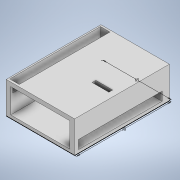
# Autodesk Inventor part: rpi case 4
Saved by Autodesk Inventor 2022.1 (Build 261234020, 234B)
## iProperties
Created: 2022-01-29
Part Number: rpi case 4
Material: Generic
Document SubType Name: Modeling
Designer: 46734
Density: 1 g/cm^3
Appearance: Default
Author: 46734
Autodesk Inventor part; units mm, degrees
ref_plane "YZ Plane" through (0, 0, 0) normal (1, 0, 0) x (0, 1, 0)
ref_plane "XZ Plane" through (0, 0, 0) normal (0, 1, 0) x (-1, 0, 0)
ref_plane "XY Plane" through (0, 0, 0) normal (0, 0, 1) x (1, 0, 0)
sketch "Sketch1" plane through (0, 0, 0) normal (0, 1, 0) x (-1, 0, 0)
  line L0 (32.5, 45) -> (-32.5, 45)
  line L1 (-32.5, 45) -> (-32.5, -45)
  line L2 (-32.5, -45) -> (32.5, -45)
  line L3 (32.5, -45) -> (32.5, 45)
  line L4 (32.5, 45) -> (-32.5, -45) construction
  line L5 (-32.5, 45) -> (32.5, -45) construction
  point P0 (0, 0)
  dimension "d0" = 65
  dimension "d1" = 90
  constraints: 12 end point, 2 midpoint, 2 parallel, 1 horizontal, 1 perpendicular
  measures "d0" distance of L2.end L1.end
  measures "d1" distance of L1.end L0.end
extrude "Extrusion1" add sketch "Sketch1" along normal blind 30
sketch "Sketch2" plane through (0, 30, 0) normal (0, 1, 0) x (1, 0, 0)
  line L0 (-31.1199, -43.0237) -> (-22.1071, -43.0237)
  line L1 (-22.1071, -43.0237) -> (-22.1071, 43.1938)
  line L2 (-22.1071, 43.1938) -> (-31.1199, 43.1938)
  line L3 (-31.1199, 43.1938) -> (-31.1199, -43.0237)
  point P0 (0, 0)
  constraints: 8 end point, 2 parallel, 1 horizontal, 1 perpendicular
extrude "Extrusion2" cut sketch "Sketch2" against normal blind 10
sketch "Sketch3" plane through (-32.5, 0, 45) normal (0, 0, 1) x (1, 0, 0)
  line L0 (4.271, 2.8909) -> (60.559, 2.8909)
  line L1 (60.559, 2.8909) -> (60.559, 26.1884)
  line L2 (60.559, 26.1884) -> (4.271, 26.1884)
  line L3 (4.271, 26.1884) -> (4.271, 2.8909)
  point P0 (32.5, 0)
  constraints: 8 end point, 2 parallel, 1 horizontal, 1 perpendicular
extrude "Extrusion3" cut sketch "Sketch3" against normal blind 30
sketch "Sketch4" plane through (32.5, 0, 45) normal (1, 0, 0) x (0, 0, -1)
  line L0 (0, 2.8909) -> (30, 2.8909) projected
  line L1 (3.6768, 2.8909) -> (83.0922, 2.8909)
  line L2 (83.0922, 2.8909) -> (83.0922, 11.2236)
  line L3 (83.0922, 11.2236) -> (3.6768, 11.2236)
  line L4 (3.6768, 11.2236) -> (3.6768, 2.8909)
  point P0 (45, 0)
  constraints: 8 end point, 2 parallel, 1 horizontal, 1 perpendicular, 1 point on line
extrude "Extrusion4" cut sketch "Sketch4" against normal blind 30
sketch "Sketch5" plane through (0, 30, 0) normal (0, 1, 0) x (1, 0, 0)
  line L0 (26.8686, -6.8022) -> (10.8835, -6.8022)
  line L1 (10.8835, -6.8022) -> (10.8835, -3.231)
  line L2 (10.8835, -3.231) -> (26.8686, -3.231)
  line L3 (26.8686, -3.231) -> (26.8686, -6.8022)
  point P0 (0, 0)
  constraints: 8 end point, 2 parallel, 1 horizontal, 1 perpendicular
extrude "Extrusion5" cut sketch "Sketch5" against normal blind 10
body "Solid1"
